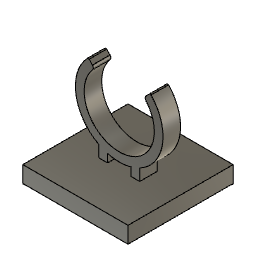
12mm hose side holder (Autodesk Fusion 360 design; units mm, degrees)
Autodesk Fusion 360 part; units mm, degrees
sketch "Sketch1" plane through (0, 0, 0) normal (0, 0, 1) x (1, 0, 0)
  line L0 (9, 9) -> (-9, 9)
  line L1 (-9, 9) -> (-9, -9)
  line L2 (-9, -9) -> (9, -9)
  line L3 (9, -9) -> (9, 9)
  line L4 (9, 9) -> (-9, -9) construction
  line L5 (-9, 9) -> (9, -9) construction
  dimension "d1" = 18
  dimension "d2" = 18
  constraint horizontal L0
  constraint perpendicular L0 L1
  constraint parallel L0 L2
  constraint parallel L1 L3
  constraint coincident L4 origin
  constraint coincident L5 origin
  measures "d1" distance of L1.end L2.end
  measures "d2" distance of L0.end L1.end
extrude "Extrude1" add sketch "Sketch1" along normal blind 3
sketch "Sketch2" plane through (0, 0, 3) normal (0, 0, 1) x (-1, 0, 0)
  line L0 (-9, 9) -> (-9, -9)
  line L1 (-9, -9) -> (9, -9)
  line L2 (9, -9) -> (9, 9)
  line L3 (9, 9) -> (-9, 9)
  line L4 (2, -1.5) -> (3.5, -1.5)
  line L5 (3.5, -1.5) -> (3.5, 1.5)
  line L6 (3.5, 1.5) -> (2, 1.5)
  line L7 (2, 1.5) -> (2, -1.5)
  line L8 (2, -1.5) -> (3.5, 1.5) construction
  line L9 (3.5, -1.5) -> (2, 1.5) construction
  line L10 (-3.5, -1.5) -> (-2, -1.5)
  line L11 (-2, -1.5) -> (-2, 1.5)
  line L12 (-2, 1.5) -> (-3.5, 1.5)
  line L13 (-3.5, 1.5) -> (-3.5, -1.5)
  line L14 (-3.5, -1.5) -> (-2, 1.5) construction
  line L15 (-2, -1.5) -> (-3.5, 1.5) construction
  line L16 (0, -12) -> (0, 14) construction
  point P0 (2.75, 0)
  point P1 (-2.75, 0)
  dimension "d5" = 3
  dimension "d6" = 1.5
  dimension "d7" = 1.5
  dimension "d8" = 3
  dimension "d9" = 2
  constraint horizontal L4
  constraint perpendicular L4 L5
  constraint parallel L4 L6
  constraint parallel L5 L7
  constraint coincident L8 P0
  constraint coincident L9 P0
  constraint horizontal L10
  constraint perpendicular L10 L11
  constraint parallel L10 L12
  constraint parallel L11 L13
  constraint coincident L14 P1
  constraint coincident L15 P1
  constraint vertical L16
  constraint symmetric P0 P1 L16
  measures "d5" distance of L4.end L5.end
  measures "d6" distance of L5.end L6.end
  measures "d7" distance of L11.end L12.end
  measures "d8" distance of L10.end L11.end
  measures "d9" distance of L7 L16
extrude "Extrude2" add sketch "Sketch2" along normal blind 2 contours L4 L5 L6 L7 | L10 L11 L12 L13
sketch "Sketch8" plane through (0, 1.5, 0) normal (0, 1, 0) x (-1, 0, 0)
  line L0 (-3.5, 3) -> (-2, 3)
  line L1 (-2, 3) -> (-2, 5)
  line L2 (-2, 5) -> (-3.5, 5)
  line L3 (-3.5, 5) -> (-3.5, 3)
  line L4 (-4.2426, 15.8759) -> (-5.3033, 16.9366)
  line L5 (0, 11.6332) -> (7.5, 11.6332) construction
  line L6 (4.2426, 15.8759) -> (5.3033, 16.9366)
  arc A0 (-5.3033, 16.9366) -> (5.3033, 16.9366) centre (0, 11.6332) ccw
  arc A1 (-4.2426, 15.8759) -> (4.2426, 15.8759) centre (0, 11.6332) ccw
  point P0 (3.5, 5)
  dimension "d18" = 15
  dimension "d19" = 12
  dimension "d20" = 135
  constraint coincident L2.end A0
  constraint coincident P0 A0
  constraint concentric A0 A1
  constraint horizontal L5
  constraint coincident L5.start A0.centre
  constraint perpendicular L4 L6
  measures "d18" diameter of A0
  measures "d19" diameter of A1
  measures "d20" angle of L4 L5
extrude "Extrude3" add 1 faces at (-2.5, 1.5, 3.6667) along direction (0, -1, 0) blind 3
extrude "Extrude4" add sketch "Sketch8" against normal blind 3 contours L1 L2 L4 L6 A0 A1
fillet "Fillet1" radius 0.5 2 edges at (-4.2426, 0, 15.8759) (4.2426, 0, 15.8759)
fillet "Fillet2" radius 0.2 4 edges at (9, 0, 0) (0, 9, 0) (-9, 0, 0) (0, -9, 0)
fillet "Fillet3" radius 0.2 2 edges at (5.3033, 0, 16.9366) (-5.3033, 0, 16.9366)
